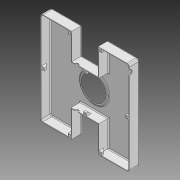
# Autodesk Inventor part: Lid
Saved by Autodesk Inventor 2020 (Build 240168000, 168)
## iProperties
Created: 2020-11-03
Part Number: Lid
Material: Generic
Document SubType Name: Modeling
Designer: DDeGo
Density: 1 g/cm^3
Appearance: Default
Author: DDeGo
Autodesk Inventor part; units mm, degrees
ref_plane "YZ Plane" through (0, 0, 0) normal (1, 0, 0) x (0, 1, 0)
ref_plane "XZ Plane" through (0, 0, 0) normal (0, 1, 0) x (-1, 0, 0)
ref_plane "XY Plane" through (0, 0, 0) normal (0, 0, 1) x (1, 0, 0)
sketch "Sketch1" plane through (0, 0, 0) normal (0, 0, 1) x (1, 0, 0)
  line L0 (92.5, -92.5) -> (92.5, 92.5)
  line L1 (-92.5, 92.5) -> (-92.5, -92.5)
  arc A0 (-87.5, 97.5) -> (-92.5, 92.5) centre (-87.5, 92.5) ccw
  arc A1 (92.5, 92.5) -> (87.5, 97.5) centre (87.5, 92.5) ccw
  arc A2 (87.5, -97.5) -> (92.5, -92.5) centre (87.5, -92.5) ccw
  arc A3 (-92.5, -92.5) -> (-87.5, -97.5) centre (-87.5, -92.5) ccw
  line L2 (-27.5, 97.5) -> (-27.5, 42.5)
  line L3 (-27.5, 42.5) -> (27.5, 42.5)
  line L4 (27.5, 42.5) -> (27.5, 97.5)
  line L5 (-27.5, -97.5) -> (-27.5, -42.5)
  line L6 (-27.5, -42.5) -> (27.5, -42.5)
  line L7 (27.5, -42.5) -> (27.5, -97.5)
  line L8 (87.5, 97.5) -> (27.5, 97.5)
  line L9 (-27.5, 97.5) -> (-87.5, 97.5)
  line L10 (-87.5, -97.5) -> (-27.5, -97.5)
  line L11 (27.5, -97.5) -> (87.5, -97.5)
  line L12 (92.5, 0) -> (-92.5, 0) construction
  point P0 (0, 0)
  point P1 (0, 0)
  dimension "d0" = 5
  dimension "d1" = 185
  dimension "d5" = 195
  dimension "d6" = 55
  dimension "d7" = 55
  constraints: 26 end point, 12 tangent, 8 point on circle, 7 parallel, 6 perpendicular, 4 centre point, 4 equal length, 3 equal radius, 3 midpoint, 2 horizontal, 1 coincident
  measures "d0" radius of A0
  measures "d1" distance between parallel lines of L0 L1
  measures "d5" distance between parallel lines of L9 L10
  measures "d6" distance of L2.end L3.end
  measures "d7" distance of L3.end L4.end
extrude "Extrusion1" add sketch "Sketch1" along normal blind 1
sketch "Sketch2" plane through (0, 0, 1) normal (0, 0, 1) x (1, 0, 0)
  line L0 (-92.5, 92.5) -> (-92.5, -92.5) projected
  arc A0 (-92.5, -92.5) -> (-87.5, -97.5) centre (-87.5, -92.5) ccw projected
  line L1 (-87.5, -97.5) -> (-27.5, -97.5) projected
  line L2 (-27.5, -97.5) -> (-27.5, -42.5) projected
  line L3 (-27.5, -42.5) -> (27.5, -42.5) projected
  line L4 (27.5, -42.5) -> (27.5, -97.5) projected
  line L5 (27.5, -97.5) -> (87.5, -97.5) projected
  arc A1 (87.5, -97.5) -> (92.5, -92.5) centre (87.5, -92.5) ccw projected
  line L6 (92.5, -92.5) -> (92.5, 92.5) projected
  arc A2 (92.5, 92.5) -> (87.5, 97.5) centre (87.5, 92.5) ccw projected
  line L7 (87.5, 97.5) -> (27.5, 97.5) projected
  line L8 (27.5, 97.5) -> (27.5, 42.5) projected
  line L9 (27.5, 42.5) -> (-27.5, 42.5) projected
  line L10 (-27.5, 42.5) -> (-27.5, 97.5) projected
  line L11 (-27.5, 97.5) -> (-87.5, 97.5) projected
  arc A3 (-87.5, 97.5) -> (-92.5, 92.5) centre (-87.5, 92.5) ccw projected
  line L12 (91, 92.5) -> (91, -92.5)
  arc A4 (87.5, -96) -> (91, -92.5) centre (87.5, -92.5) ccw
  line L13 (87.5, -96) -> (29, -96)
  line L14 (29, -96) -> (29, -41)
  line L15 (29, -41) -> (-29, -41)
  line L16 (-29, -41) -> (-29, -96)
  line L17 (-29, -96) -> (-87.5, -96)
  arc A5 (-91, -92.5) -> (-87.5, -96) centre (-87.5, -92.5) ccw
  line L18 (-91, -92.5) -> (-91, 92.5)
  arc A6 (-87.5, 96) -> (-91, 92.5) centre (-87.5, 92.5) ccw
  line L19 (-87.5, 96) -> (-29, 96)
  line L20 (-29, 96) -> (-29, 41)
  line L21 (-29, 41) -> (29, 41)
  line L22 (29, 41) -> (29, 96)
  line L23 (29, 96) -> (87.5, 96)
  arc A7 (91, 92.5) -> (87.5, 96) centre (87.5, 92.5) ccw
  point P0 (0, 0)
  dimension "d8" = 1.5
  constraints: 24 end point, 8 point on circle, 4 centre point, 15 other
  measures "d8" distance between parallel lines of L12 L6
extrude "Extrusion2" add sketch "Sketch2" along normal blind 20
sketch "Sketch3" plane through (-27.5, 42.5, 0) normal (0, 1, 0) x (1, 0, 0)
  line L0 (0, -21) -> (55, -21) projected
  circle A0 centre (10, -21) radius 4
  line L1 (0, 0) -> (0, -21) projected
  point P0 (27.5, 0)
  point P1 (14, -21)
  point P2 (6, -21)
  dimension "d11" = 8
  dimension "d12" = 10
  constraints: 1 centre point, 1 point on line
  measures "d11" diameter of A0
  measures "d12" distance from line of L1 A0.centre
extrude "Extrusion3" cut sketch "Sketch3" against normal blind 91 contours A0 L0 picked at (10.1607, -19.6764)
fillet "Fillet1" radius 2 32 edges at (-89.9749, -94.9749, 1) (-58.25, -96, 1) (-89.9749, 94.9749, 1) (-58.25, 96, 1) (-91, 0, 1) (89.9749, 94.9749, 1) (91, 0, 1) (89.9749, -94.9749, 1) (58.25, -96, 1) (58.25, 96, 1) (29, 68.5, 1) (0, 41, 1) (-29, 68.5, 1) (-29, -68.5, 1) (0, -41, 1) (29, -68.5, 1) (-92.5, 0, 0) (-91.0355, -96.0355, 0) (-57.5, -97.5, 0) (-57.5, 97.5, 0) (-91.0355, 96.0355, 0) (-27.5, 70, 0) (0, 42.5, 0) (0, -42.5, 0) (-27.5, -70, 0) (27.5, -70, 0) (91.0355, -96.0355, 0) (92.5, 0, 0) (91.0355, 96.0355, 0) (57.5, 97.5, 0) (57.5, -97.5, 0) (27.5, 70, 0)
sketch "Sketch4" plane through (0, 0, 21) normal (0, 0, 1) x (1, 0, 0)
  line L0 (87.5, -96) -> (29, -96) construction
  line L1 (91, 92.5) -> (91, -92.5) construction
  line L2 (0, 0) -> (0, 41) construction
  line L3 (29, 96) -> (87.5, 96) construction
  line L4 (29, 41) -> (29, 96) construction
  line L5 (29, 96) -> (35, 96)
  line L6 (35, 96) -> (35, 90)
  line L7 (35, 90) -> (29, 90)
  line L8 (29, 90) -> (29, 96)
  line L9 (35, 90) -> (29, 96) construction
  circle A0 centre (32, 93) radius 1.5
  line L10 (29, -96) -> (29, -41) construction
  line L11 (29, -96) -> (35, -96)
  line L12 (35, -96) -> (35, -90)
  line L13 (35, -90) -> (29, -90)
  line L14 (29, -90) -> (29, -96)
  line L15 (29, -96) -> (31, -94) projected
  line L16 (29, -96) -> (35, -90) construction
  circle A1 centre (32, -93) radius 1.5
  line L17 (0, 0) -> (0, -41) construction
  line L18 (29, -41) -> (-13.5, -41) construction
  line L19 (-13.5, 41) -> (29, 41) construction
  line L20 (-3, -35) -> (3, -35)
  line L21 (3, -35) -> (3, -41)
  line L22 (3, -41) -> (-3, -41)
  line L23 (-3, -41) -> (-3, -35)
  line L24 (-3, -35) -> (3, -41) construction
  line L25 (3, -35) -> (-3, -41) construction
  line L26 (-3, 35) -> (3, 35)
  line L27 (3, 35) -> (3, 41)
  line L28 (3, 41) -> (-3, 41)
  line L29 (-3, 41) -> (-3, 35)
  line L30 (-3, 35) -> (3, 41) construction
  line L31 (3, 35) -> (-3, 41) construction
  circle A2 centre (0, -38) radius 1.5
  circle A3 centre (0, 38) radius 1.5
  line L32 (91, 0) -> (88, 0) construction
  line L33 (85, 3) -> (91, 3)
  line L34 (91, 3) -> (91, -3)
  line L35 (91, -3) -> (85, -3)
  line L36 (85, -3) -> (85, 3)
  line L37 (85, 3) -> (91, -3) construction
  line L38 (91, 3) -> (85, -3) construction
  circle A4 centre (88, 0) radius 1.5
  line L39 (-87.5, -96) -> (-29, -96) construction
  line L40 (-91, 92.5) -> (-91, -92.5) construction
  line L41 (-29, 96) -> (-87.5, 96) construction
  line L42 (-29, 41) -> (-29, 96) construction
  line L43 (-29, 96) -> (-35, 96)
  line L44 (-35, 96) -> (-35, 90)
  line L45 (-35, 90) -> (-29, 90)
  line L46 (-29, 90) -> (-29, 96)
  line L47 (-35, 90) -> (-29, 96) construction
  circle A5 centre (-32, 93) radius 1.5
  line L48 (-29, -96) -> (-29, -41) construction
  line L49 (-29, -96) -> (-35, -96)
  line L50 (-35, -96) -> (-35, -90)
  line L51 (-35, -90) -> (-29, -90)
  line L52 (-29, -90) -> (-29, -96)
  line L53 (-29, -96) -> (-31, -94)
  line L54 (-29, -96) -> (-35, -90) construction
  circle A6 centre (-32, -93) radius 1.5
  line L55 (-29, -41) -> (13.5, -41) construction
  line L56 (13.5, 41) -> (-29, 41) construction
  line L57 (3, -35) -> (-3, -35)
  line L58 (-3, -35) -> (-3, -41)
  line L59 (-3, -41) -> (3, -41)
  line L60 (3, -41) -> (3, -35)
  line L61 (3, -35) -> (-3, -41) construction
  line L62 (-3, -35) -> (3, -41) construction
  line L63 (3, 35) -> (-3, 35)
  line L64 (-3, 35) -> (-3, 41)
  line L65 (-3, 41) -> (3, 41)
  line L66 (3, 41) -> (3, 35)
  line L67 (3, 35) -> (-3, 41) construction
  line L68 (-3, 35) -> (3, 41) construction
  circle A7 centre (0, -38) radius 1.5
  circle A8 centre (0, 38) radius 1.5
  line L69 (-91, 0) -> (-88, 0) construction
  line L70 (-85, 3) -> (-91, 3)
  line L71 (-91, 3) -> (-91, -3)
  line L72 (-91, -3) -> (-85, -3)
  line L73 (-85, -3) -> (-85, 3)
  line L74 (-85, 3) -> (-91, -3) construction
  line L75 (-91, 3) -> (-85, -3) construction
  circle A9 centre (-88, 0) radius 1.5
  dimension "d23" = 6
  dimension "d24" = 3
  constraints: 136 end point, 34 symmetric about line, 13 midpoint, 11 point on line, 10 centre point, 10 parallel, 9 equal length, 6 horizontal, 6 perpendicular, 5 coincident, 4 equal radius, 1 vertical, 5 other
  measures "d23" distance of L6.end L7.end
  measures "d24" diameter of A0
extrude "Extrusion4" add sketch "Sketch4" against normal blind 10
chamfer "Chamfer2" distance 6 angle 45 8 edges at (85, 0, 11) (0, -35, 11) (-35, -93, 11) (-35, 93, 11) (-85, 0, 11) (0, 35, 11) (35, -93, 11) (35, 93, 11)
sketch "Sketch5" plane through (0, 0, 0) normal (0, 1, 0) x (-1, 0, 0)
  line L0 (0, 0) -> (29, 0)
  line L1 (29, 0) -> (26.1601, 2.8399)
  line L2 (26.1601, 2.8399) -> (0, 2.8399)
  line L3 (0, 2.8399) -> (0, 0)
  dimension "d28" = 45
  dimension "d29" = 29
  constraints: 8 end point, 1 horizontal, 1 parallel, 1 perpendicular
  measures "d28" angle of L0 L1
  measures "d29" distance of L0.start L0.end
revolve "Revolution1" cut sketch "Sketch5" angle 360 about axis through (0, 0, 2.8399) along (0, 0, -1)
sketch "Sketch6" plane through (0, 0, 0) normal (0, 1, 0) x (-1, 0, 0)
  line L0 (28, 1) -> (26, 3)
  line L1 (26, 3) -> (29, 3)
  line L2 (35, 21) -> (35, 17) projected
  line L3 (29, 3) -> (31, 1)
  line L4 (31, 1) -> (28, 1)
  line L5 (0, 1) -> (0, 8.3076) construction
  line L6 (-28, 1) -> (28, 1) construction
  point P0 (0, 0)
  dimension "d32" = 2
  dimension "d33" = 3
  dimension "d35" = 45
  constraints: 10 end point, 2 parallel, 1 collinear
  measures "d32" distance between parallel lines of L4 L1
  measures "d33" distance of L0.start L3.end
  measures "d35" angle of L6 L0
revolve "Revolution2" add sketch "Sketch6" angle 360 about axis through (0, 0, 1) along (0, 0, 1)
fillet "Fillet2" radius 2 2 edges at (31, 0, 1) (29, 0, 3)
sketch "Sketch7" plane through (92.5, -92.5, 21) normal (1, 0, 0) x (0, 0, -1)
  line L0 (0, 185) -> (0, 0) projected
  line L1 (0, 172.5) -> (0, 167.5) construction
  line L2 (0, 190) -> (0, 135) projected
  line L3 (-7, 172.5) -> (-7, 167.5)
  line L4 (7, 167.5) -> (7, 172.5)
  arc A0 (7, 172.5) -> (-7, 172.5) centre (0, 172.5) ccw
  arc A1 (-7, 167.5) -> (7, 167.5) centre (0, 167.5) ccw
  point P0 (21, 92.5)
  point P1 (0, 170)
  point P2 (0, 179.5)
  point P3 (0, 160.5)
  dimension "d41" = 7
  dimension "d42" = 5
  dimension "d43" = 15
  constraints: 8 end point, 4 point on circle, 4 tangent, 2 centre point, 2 point on line, 1 midpoint, 1 parallel
  measures "d41" radius of A1
  measures "d42" distance of L4.start L4.end
  measures "d43" distance of L0.start point (0, 170)
extrude "Extrusion5" cut sketch "Sketch7" against normal blind 10 contours A0 L4 A1 L0
body "Solid1"
